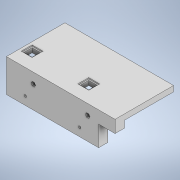
# Autodesk Inventor part: side_bumper
Saved by Autodesk Inventor 2020 (Build 240168000, 168)
## iProperties
Created: 2022-07-15
Part Number: side_bumper
Material: 일반
Document SubType Name: Modeling
Designer: SeungJin
Density: 1 g/cm^3
Appearance: 기본값
Author: SeungJin
Autodesk Inventor part; units mm, degrees
ref_plane "YZ Plane" through (0, 0, 0) normal (1, 0, 0) x (0, 1, 0)
sketch "스케치1" plane through (0, 0, 0) normal (0, 0, 1) x (1, 0, 0)
  line L0 (6, 0) -> (18, 0) projected
  line L1 (6, 0) -> (6, -540) projected
  line L2 (18, -540) -> (6, -540) projected
  line L3 (18, 0) -> (18, -540) projected
  line L4 (-12, 0) -> (0, 0) projected
  line L5 (-12, 0) -> (-12, -540) projected
  line L6 (0, -540) -> (-12, -540) projected
  line L7 (0, 0) -> (0, -540) projected
  line L8 (18, 22.5444) -> (18, 12.5098) projected
  line L9 (18, 12.5098) -> (18, -220) projected
  line L10 (-192.5399, 0) -> (-180.5399, 0) projected
  line L11 (-192.5399, 0) -> (-192.5399, -540) projected
  line L12 (-180.5399, -540) -> (-192.5399, -540) projected
  line L13 (-180.5399, 0) -> (-180.5399, -540) projected
  line L14 (-210.5399, 0) -> (-198.5399, 0) projected
  line L15 (-210.5399, 0) -> (-210.5399, -540) projected
  line L16 (-198.5399, -540) -> (-210.5399, -540) projected
  line L17 (-198.5399, 0) -> (-198.5399, -540) projected
  line L18 (18, 22.5444) -> (-210.5399, 22.5444)
  line L19 (-210.5399, 22.5444) -> (-210.5399, -37.4556)
  line L20 (-210.5399, -37.4556) -> (18, -37.4556)
  line L21 (18, -37.4556) -> (18, 22.5444)
  line L22 (18, 12.5444) -> (-210.5399, 12.5444)
  dimension "d0" = 60
  dimension "d1" = 10
  constraints: 10 end point, 3 point on line, 2 parallel, 2 perpendicular, 1 horizontal
  measures "d0" distance of L19.end L18.end
  measures "d1" distance between parallel lines of L22 L18
extrude "돌출1" add sketch "스케치1" along normal blind 10 and the other way blind 150 contours L22 L19 L18 L8
sketch "스케치2" plane through (-210.5399, 22.5444, 10) normal (0, 1, 0) x (1, 0, 0)
  line L0 (0, 0) -> (0, 160) projected
  line L1 (228.5399, 0) -> (0, 0) projected
  line L2 (228.5399, 160) -> (228.5399, 0) projected
  line L3 (0, 160) -> (228.5399, 160) projected
  circle A0 centre (-63.5, 111.3) radius 75.8469 projected
  line L4 (-155.5399, 160) -> (-155.5399, 55) projected
  line L5 (-139.3469, 111.3) -> (-155.5399, 111.3)
  line L6 (0, 0) -> (228.5399, 0) projected
  line L7 (30, 0) -> (30, 160)
  line L8 (0, 160) -> (0, 0) projected
  line L9 (30, 0) -> (0, 0)
  line L10 (0, 0) -> (0, 40)
  line L11 (0, 40) -> (30, 40)
  line L12 (30, 40) -> (30, 0)
  point P0 (210.5399, 10)
  point P1 (30, 40)
  dimension "d7" = 16.193
  dimension "d8" = 40
  dimension "d44" = 30
  constraints: 12 end point, 4 point on line, 3 perpendicular, 2 parallel, 1 horizontal, 1 horizontal alignment, 1 other
  measures "d7" distance of L5.start L5.end
  measures "d8" distance of L9.end L10.end
  measures "d44" distance between parallel lines of L7 L0
extrude "돌출2" cut sketch "스케치2" against normal through all contours L0 A0 L3 L7 L11 | L0 A0 picked at (1.772, 100.6693)
ref_plane "작업 평면1" through (-180.5399, 0, 0) normal (0, 0, 1) x (1, 0, 0)
sketch "스케치3" plane through (-180.5399, 0, 0) normal (0, 0, 1) x (1, 0, 0)
  line L0 (-30, 22.5444) -> (-30, 12.5444) projected
  line L1 (-30, 12.5444) -> (198.5399, 12.5444) projected
  line L2 (198.5399, 12.5444) -> (198.5399, 22.5444) projected
  line L3 (198.5399, 22.5444) -> (-30, 22.5444) projected
  line L4 (-30, 12.5444) -> (198.5399, 12.5444) projected
  line L5 (-30, 0) -> (-18, 0) projected
  line L6 (-30, 0) -> (-30, -540) projected
  line L7 (-18, -540) -> (-30, -540) projected
  line L8 (-18, 0) -> (-18, -540) projected
  line L9 (-12, 0) -> (0, 0) projected
  line L10 (-12, 0) -> (-12, -540) projected
  line L11 (0, -540) -> (-12, -540) projected
  line L12 (0, 0) -> (0, -540) projected
  line L13 (168.5399, 0) -> (180.5399, 0) projected
  line L14 (168.5399, 0) -> (168.5399, -540) projected
  line L15 (180.5399, -540) -> (168.5399, -540) projected
  line L16 (180.5399, 0) -> (180.5399, -540) projected
  line L17 (186.5399, 0) -> (198.5399, 0) projected
  line L18 (186.5399, 0) -> (186.5399, -540) projected
  line L19 (198.5399, -540) -> (186.5399, -540) projected
  line L20 (198.5399, 0) -> (198.5399, -540) projected
  line L21 (198.5399, 12.5444) -> (-30, 12.5444)
  line L22 (-30, 12.5444) -> (-30, -37.4556)
  line L23 (-30, -37.4556) -> (198.5399, -37.4556)
  line L24 (198.5399, -37.4556) -> (198.5399, 12.5444)
  dimension "d11" = 50
  constraints: 8 end point, 2 parallel, 1 horizontal, 1 perpendicular, 1 point on line
  measures "d11" distance of L22.end L21.end
extrude "돌출3" add sketch "스케치3" along normal blind 10 contours L1 L24 L17 L18 L23 L16 L13 L14 L12 L9 L10 L8 L5 L22 | L5 L8 L23 L6 | L20 L23 L18 L17 | L10 L9 L12 L23 | L23 L14 L13 L16
ref_plane "작업 평면2" through (-12, -260, -30) normal (0, 0, -1) x (0, 1, 0)
sketch "스케치4" plane through (-180.5399, 0, 0) normal (0, 0, -1) x (-1, 0, 0)
  line L0 (-180.5399, -260) -> (-168.5399, -260)
  line L1 (-168.5399, 0) -> (-168.5399, -260)
  line L2 (-180.5399, 0) -> (-168.5399, 0)
  line L3 (-180.5399, 0) -> (-180.5399, -260)
  line L4 (-198.5399, -260) -> (-186.5399, -260)
  line L5 (-186.5399, 0) -> (-186.5399, -260)
  line L6 (-198.5399, 0) -> (-186.5399, 0)
  line L7 (-198.5399, 0) -> (-198.5399, -260)
  line L8 (0, 12.5444) -> (0, 22.5444)
  line L9 (0, 22.5444) -> (-198.5399, 22.5444)
  line L10 (-198.5399, 22.5444) -> (-198.5399, 12.5444)
  line L11 (-198.5399, 12.5444) -> (0, 12.5444)
  line L12 (30, 12.5444) -> (0, 12.5444)
  line L13 (30, 22.5444) -> (30, 12.5444)
  line L14 (0, 22.5444) -> (30, 22.5444)
  line L15 (0, 22.5444) -> (0, 12.5444)
  line L16 (18, -260) -> (30, -260)
  line L17 (30, 0) -> (30, -260)
  line L18 (18, 0) -> (30, 0)
  line L19 (18, 0) -> (18, -260)
  line L20 (0, -260) -> (12, -260)
  line L21 (12, 0) -> (12, -260)
  line L22 (0, 0) -> (12, 0)
  line L23 (0, 0) -> (0, -260)
  line L24 (-198.5399, 0) -> (30, 0)
  line L25 (30, 0) -> (30, 12.5444)
  line L26 (30, 12.5444) -> (-198.5399, 12.5444)
  line L27 (-198.5399, 12.5444) -> (-198.5399, 0)
  line L28 (30, 12.5444) -> (30, -37.4556)
  line L29 (-198.5399, 12.5444) -> (30, 12.5444)
  line L30 (-198.5399, -37.4556) -> (-198.5399, 12.5444)
  line L31 (30, -37.4556) -> (-198.5399, -37.4556)
  line L32 (-198.5399, 0) -> (30, 0)
  line L33 (30, 0) -> (30, -37.4556)
  line L34 (30, -37.4556) -> (-198.5399, -37.4556)
  line L35 (-198.5399, -37.4556) -> (-198.5399, 0)
  line L36 (30, -37.4556) -> (-198.5399, -37.4556)
  line L37 (-99.27, 0) -> (-69.27, 0)
  line L38 (-69.27, 0) -> (-69.27, -37.4556)
  line L39 (-69.27, -37.4556) -> (-99.27, -37.4556)
  line L40 (-99.27, -37.4556) -> (-99.27, 0)
  line L41 (-99.27, 0) -> (-69.27, -37.4556) construction
  line L42 (-69.27, 0) -> (-99.27, -37.4556) construction
  line L43 (0, 0) -> (0, 12.5444)
  point P0 (-84.27, -18.7278)
  point P1 (0, -37.4556)
  point P2 (-168.5399, -37.4556)
extrude "돌출4" add sketch "스케치4" along normal blind 60 contours L1 L24 L40 L31 | L24 L6 L27 L11 L43 L2 | L40 L24 L38 L31 | L38 L24 L23 L31
sketch "스케치7" plane through (-180.5399, 0, 0) normal (0, 0, -1) x (-1, 0, 0)
  line L0 (0, -260) -> (12, -260) projected
  line L1 (12, 0) -> (12, -260) projected
  line L2 (0, 0) -> (12, 0) projected
  line L3 (0, 0) -> (0, -260) projected
  line L4 (18, -260) -> (30, -260) projected
  line L5 (30, 0) -> (30, -260) projected
  line L6 (18, 0) -> (30, 0) projected
  line L7 (18, 0) -> (18, -260) projected
  line L8 (30, 12.5444) -> (0, 12.5444) projected
  line L9 (30, 22.5444) -> (30, 12.5444) projected
  line L10 (0, 22.5444) -> (30, 22.5444) projected
  line L11 (0, 22.5444) -> (0, 12.5444) projected
  line L12 (-198.5399, 12.5444) -> (0, 12.5444) projected
  line L13 (0, 12.5444) -> (30, 12.5444)
  line L14 (30, 12.5444) -> (30, 0)
  line L15 (30, 0) -> (0, 0)
  line L16 (0, 0) -> (0, 12.5444)
  point P0 (-180.5399, 0)
  constraints: 8 end point, 2 parallel, 1 horizontal, 1 perpendicular
extrude "돌출7" add sketch "스케치7" along normal blind 30 contours L16 L8 L14 L6 L15 L2
sketch "스케치9" plane through (-210.5399, 22.5444, 10) normal (0, 1, 0) x (1, 0, 0)
  line L0 (30, 40) -> (0, 40) projected
  line L1 (0, 0) -> (0, 40) projected
  line L2 (228.5399, 0) -> (0, 0) projected
  line L3 (228.5399, 160) -> (228.5399, 0) projected
  line L4 (30, 160) -> (228.5399, 160) projected
  line L5 (30, 160) -> (30, 40) projected
  line L6 (30, 160) -> (30, 40) projected
  line L7 (228.5399, 75) -> (30, 75)
  line L8 (30, 75) -> (30, 95)
  line L9 (30, 95) -> (228.5399, 95)
  line L10 (228.5399, 95) -> (228.5399, 75)
  line L11 (158.5399, 75) -> (138.5399, 75)
  line L12 (138.5399, 75) -> (138.5399, 95)
  line L13 (138.5399, 95) -> (158.5399, 95)
  line L14 (158.5399, 95) -> (158.5399, 75)
  line L15 (158.5399, 75) -> (138.5399, 95) construction
  line L16 (138.5399, 75) -> (158.5399, 95) construction
  line L17 (55, 75) -> (35, 75)
  line L18 (35, 75) -> (35, 95)
  line L19 (35, 95) -> (55, 95)
  line L20 (55, 95) -> (55, 75)
  line L21 (55, 75) -> (35, 95) construction
  line L22 (35, 75) -> (55, 95) construction
  point P0 (210.5399, 10)
  point P1 (148.5399, 85)
  point P2 (45, 85)
  point P3 (55, 75)
  point P4 (55, 95)
  point P5 (35, 75)
  point P6 (158.5399, 75)
  point P7 (138.5399, 75)
  point P8 (148.5399, 85)
  point P9 (228.5399, 85)
  point P10 (45, 85)
  point P11 (30, 85)
  dimension "d45" = 20
  dimension "d46" = 65
  dimension "d48" = 80
  dimension "d49" = 20
  dimension "d50" = 15
  dimension "d101" = 20
  constraints: 32 end point, 8 midpoint, 6 parallel, 4 point on line, 3 horizontal, 3 perpendicular, 2 horizontal alignment
  measures "d45" distance of L7.end L8.end
  measures "d46" distance between parallel lines of L4 L9
  measures "d48" distance from line of point (148.54, 85) L3
  measures "d49" distance of L18.end L19.end
  measures "d50" distance from line of L5 point (45, 85)
  measures "d101" distance of L11.start L11.end
extrude "돌출8" cut sketch "스케치9" against normal blind 2 contours L18 L9 L20 L7 | L12 L9 L14 L7
sketch "스케치10" plane through (-210.5399, 20.5444, 10) normal (0, 1, 0) x (1, 0, 0)
  line L0 (138.5399, 75) -> (138.5399, 95) projected
  line L1 (158.5399, 75) -> (138.5399, 75) projected
  line L2 (158.5399, 95) -> (158.5399, 75) projected
  line L3 (138.5399, 95) -> (158.5399, 95) projected
  line L4 (55, 75) -> (35, 75) projected
  line L5 (55, 95) -> (55, 75) projected
  line L6 (35, 95) -> (55, 95) projected
  line L7 (35, 75) -> (35, 95) projected
  line L8 (156.0399, 77.5) -> (141.0399, 77.5)
  line L9 (141.0399, 77.5) -> (141.0399, 92.5)
  line L10 (141.0399, 92.5) -> (156.0399, 92.5)
  line L11 (156.0399, 92.5) -> (156.0399, 77.5)
  line L12 (156.0399, 77.5) -> (141.0399, 92.5) construction
  line L13 (141.0399, 77.5) -> (156.0399, 92.5) construction
  line L14 (52.5, 77.5) -> (37.5, 77.5)
  line L15 (37.5, 77.5) -> (37.5, 92.5)
  line L16 (37.5, 92.5) -> (52.5, 92.5)
  line L17 (52.5, 92.5) -> (52.5, 77.5)
  line L18 (52.5, 77.5) -> (37.5, 92.5) construction
  line L19 (37.5, 77.5) -> (52.5, 92.5) construction
  point P0 (210.5399, 10)
  point P1 (148.5399, 85)
  point P2 (45, 85)
  dimension "d53" = 15
  dimension "d54" = 15
  dimension "d55" = 15
  dimension "d56" = 15
  constraints: 24 end point, 4 midpoint, 4 parallel, 2 horizontal, 2 perpendicular
  measures "d53" distance of L9.end L10.end
  measures "d54" distance of L8.end L9.end
  measures "d55" distance of L15.end L16.end
  measures "d56" distance of L14.end L15.end
extrude "돌출9" cut sketch "스케치10" against normal through all contours L8 L9 L10 L11 | L14 L15 L16 L17
sketch "스케치11" plane through (-180.5399, 0, -60) normal (0, 0, -1) x (-1, 0, 0)
  line L0 (0, 12.5444) -> (0, 22.5444) projected
  line L1 (0, 22.5444) -> (-198.5399, 22.5444) projected
  line L2 (-198.5399, 22.5444) -> (-198.5399, 12.5444) projected
  line L3 (-198.5399, 12.5444) -> (0, 12.5444) projected
  line L4 (-168.5399, -37.4556) -> (0, -37.4556) projected
  line L5 (-198.5399, 12.5444) -> (0, 12.5444) projected
  line L6 (-198.5399, 12.5444) -> (-198.5399, 0) projected
  line L7 (-198.5399, 0) -> (-168.5399, 0) projected
  line L8 (-168.5399, 0) -> (-168.5399, -37.4556) projected
  line L9 (0, -37.4556) -> (0, 12.5444) projected
  line L10 (-198.5399, 12.5444) -> (0, 12.5444)
  line L11 (0, 12.5444) -> (0, -5.4556)
  line L12 (0, -5.4556) -> (-198.5399, -5.4556)
  line L13 (-198.5399, -5.4556) -> (-198.5399, 12.5444)
  line L14 (-128.5399, 12.5444) -> (-108.5399, 12.5444)
  line L15 (-108.5399, 12.5444) -> (-108.5399, -5.4556)
  line L16 (-108.5399, -5.4556) -> (-128.5399, -5.4556)
  line L17 (-128.5399, -5.4556) -> (-128.5399, 12.5444)
  line L18 (-128.5399, 12.5444) -> (-108.5399, -5.4556) construction
  line L19 (-108.5399, 12.5444) -> (-128.5399, -5.4556) construction
  line L20 (-25, 12.5444) -> (-5, 12.5444)
  line L21 (-5, 12.5444) -> (-5, -5.4556)
  line L22 (-5, -5.4556) -> (-25, -5.4556)
  line L23 (-25, -5.4556) -> (-25, 12.5444)
  line L24 (-25, 12.5444) -> (-5, -5.4556) construction
  line L25 (-5, 12.5444) -> (-25, -5.4556) construction
  circle A0 centre (-34.635, -22.4556) radius 3.6
  circle A1 centre (-133.9049, -22.4556) radius 3.6
  line L26 (-36.7134, -26.0556) -> (-38.7919, -22.4556)
  line L27 (-38.7919, -22.4556) -> (-36.7134, -18.8556)
  line L28 (-36.7134, -18.8556) -> (-32.5565, -18.8556)
  line L29 (-32.5565, -18.8556) -> (-30.4781, -22.4556)
  line L30 (-30.4781, -22.4556) -> (-32.5565, -26.0556)
  line L31 (-32.5565, -26.0556) -> (-36.7134, -26.0556)
  line L32 (-135.9834, -26.0556) -> (-138.0619, -22.4556)
  line L33 (-138.0619, -22.4556) -> (-135.9834, -18.8556)
  line L34 (-135.9834, -18.8556) -> (-131.8265, -18.8556)
  line L35 (-131.8265, -18.8556) -> (-129.748, -22.4556)
  line L36 (-129.748, -22.4556) -> (-131.8265, -26.0556)
  line L37 (-131.8265, -26.0556) -> (-135.9834, -26.0556)
  line L38 (0, -37.4556) -> (0, 12.5444) projected
  point P0 (-180.5399, 0)
  point P1 (-118.5399, 3.5444)
  point P2 (-15, 3.5444)
  point P3 (-148.5399, 3.5444)
  point P4 (-49.27, 3.5444)
  point P5 (-34.635, -26.0556)
  point P6 (-133.9049, -26.0556)
  dimension "d71" = 7.2
  dimension "d59" = 18
  dimension "d60" = 20
  dimension "d61" = 20
  dimension "d63" = 80
  dimension "d64" = 20
  dimension "d69" = 15
  dimension "d72" = 7.2
  constraints: 56 end point, 6 midpoint, 6 parallel, 4 coincident, 4 point on line, 3 horizontal, 3 perpendicular, 1 centre point, 1 vertical alignment, 28 other
  measures "d59" distance of L10.end L11.end
  measures "d60" distance of L15.end L16.end
  measures "d61" distance of L21.end L22.end
  measures "d63" distance from line of L6 point (-118.54, 3.544)
  measures "d64" distance from line of point (-148.54, 3.544) L8
  measures "d69" distance from line of L4 point (-34.635, -22.456)
  measures "d72" diameter of A1
sketch "스케치12" plane through (-210.5399, 22.5444, 10) normal (0, 1, 0) x (1, 0, 0)
  line L0 (35, 95) -> (55, 95) projected
  line L1 (55, 95) -> (55, 75) projected
  line L2 (55, 75) -> (35, 75) projected
  line L3 (35, 75) -> (35, 95) projected
  line L4 (138.5399, 75) -> (138.5399, 95) projected
  line L5 (138.5399, 95) -> (158.5399, 95) projected
  line L6 (158.5399, 95) -> (158.5399, 75) projected
  line L7 (158.5399, 75) -> (138.5399, 75) projected
  line L8 (30, 40) -> (0, 40) projected
  line L9 (0, 0) -> (0, 40) projected
  line L10 (228.5399, 0) -> (0, 0) projected
  line L11 (228.5399, 160) -> (228.5399, 0) projected
  line L12 (30, 160) -> (228.5399, 160) projected
  line L13 (30, 160) -> (30, 40) projected
  line L14 (228.5399, 0) -> (0, 0)
  line L15 (0, 0) -> (0, 53)
  line L16 (0, 53) -> (228.5399, 53)
  line L17 (228.5399, 53) -> (228.5399, 0)
  point P0 (210.5399, 10)
  point P1 (228.5399, 53)
  point P2 (30, 53)
  dimension "d66" = 53
  constraints: 8 end point, 2 parallel, 1 horizontal, 1 perpendicular
  measures "d66" distance of L14.end L15.end
extrude "돌출10" cut sketch "스케치12" against normal through all contours L13 L16 L11 L10 L9 L8
extrude "돌출11" cut sketch "스케치11" against normal blind 12 contours A0 | A0 L29 L30 | A0 L28 L29 | L30 L31 A0 | A0 L27 L28 | L31 L26 A0 | A0 L26 L27 | A1 | A1 L35 L36 | A1 L34 L35 | L36 L37 A1 | A1 L33 L34 | L37 L32 A1 | A1 L32 L33
sketch "스케치13" plane through (-180.5399, 0, -48) normal (0, 0, -1) x (-1, 0, 0)
  line L0 (-36.7134, -18.8556) -> (-32.5565, -18.8556) projected
  line L1 (-38.7919, -22.4556) -> (-36.7134, -18.8556) projected
  line L2 (-36.7134, -26.0556) -> (-38.7919, -22.4556) projected
  line L3 (-32.5565, -26.0556) -> (-36.7134, -26.0556) projected
  line L4 (-30.4781, -22.4556) -> (-32.5565, -26.0556) projected
  line L5 (-32.5565, -18.8556) -> (-30.4781, -22.4556) projected
  line L6 (-135.9834, -26.0556) -> (-138.0619, -22.4556) projected
  line L7 (-131.8265, -26.0556) -> (-135.9834, -26.0556) projected
  line L8 (-129.748, -22.4556) -> (-131.8265, -26.0556) projected
  line L9 (-131.8265, -18.8556) -> (-129.748, -22.4556) projected
  line L10 (-135.9834, -18.8556) -> (-131.8265, -18.8556) projected
  line L11 (-138.0619, -22.4556) -> (-135.9834, -18.8556) projected
  point P0 (-180.5399, 0)
  point P1 (-34.635, -22.4556)
  point P2 (-133.9049, -22.4556)
hole "구멍1" at (-145.9049, -22.4556, -48) at (-46.635, -22.4556, -48) direction (0, 0, 1) diameter 4.5 end through all clearance for "Hex Head Cap Screw ISO 24017" size "M4" standard "ISO"
sketch "스케치14" plane through (-180.5399, 22.5444, -43) normal (0, 0, 1) x (1, 0, 0)
  circle A0 centre (34.635, -45) radius 2.25 projected
  circle A1 centre (133.9049, -45) radius 2.25 projected
  line L0 (168.5399, -60) -> (0, -60) projected
  line L1 (198.5399, -22.5444) -> (168.5399, -22.5444) projected
  line L2 (168.5399, -22.5444) -> (168.5399, -60) projected
  line L3 (198.5399, 0) -> (198.5399, -22.5444) projected
  line L4 (0, 0) -> (198.5399, 0) projected
  line L5 (0, -60) -> (0, 0) projected
  line L6 (0, 0) -> (198.5399, 0) projected
  line L7 (198.5399, 0) -> (198.5399, -22.5444) projected
  line L8 (0, 0) -> (198.5399, 0)
  line L9 (198.5399, 0) -> (198.5399, -22.5444)
  line L10 (0, -22.5444) -> (0, 0)
  line L11 (5, -22.5444) -> (25, -22.5444)
  line L12 (25, -22.5444) -> (25, 0)
  line L13 (25, 0) -> (5, 0)
  line L14 (5, 0) -> (5, -22.5444)
  line L15 (5, -22.5444) -> (25, 0) construction
  line L16 (25, -22.5444) -> (5, 0) construction
  line L17 (108.5399, -22.5444) -> (128.5399, -22.5444)
  line L18 (128.5399, -22.5444) -> (128.5399, 0)
  line L19 (128.5399, 0) -> (108.5399, 0)
  line L20 (108.5399, 0) -> (108.5399, -22.5444)
  line L21 (108.5399, -22.5444) -> (128.5399, 0) construction
  line L22 (128.5399, -22.5444) -> (108.5399, 0) construction
  line L23 (0, -60) -> (0, -10) projected
  line L24 (0, -28) -> (198.5399, -28)
  line L25 (0, -10) -> (198.5399, -10)
  line L26 (25, -28) -> (25, -22.5444)
  line L27 (69.27, -22.5444) -> (69.27, -60) projected
  line L28 (69.27, -28) -> (69.27, -10)
  line L29 (168.5399, -22.5444) -> (168.5399, -60) projected
  line L30 (168.5399, -28) -> (168.5399, -10)
  line L31 (128.5399, -22.5444) -> (128.5399, -28)
  line L32 (25, -22.5444) -> (0, -22.5444)
  line L33 (198.5399, -22.5444) -> (168.5399, -22.5444)
  line L34 (128.5399, -22.5444) -> (69.27, -22.5444)
  circle A2 centre (49.27, -19) radius 3.6
  circle A3 centre (148.5399, -19) radius 3.6
  line L35 (47.1915, -22.6) -> (45.113, -19)
  line L36 (45.113, -19) -> (47.1915, -15.4)
  line L37 (47.1915, -15.4) -> (51.3484, -15.4)
  line L38 (51.3484, -15.4) -> (53.4269, -19)
  line L39 (53.4269, -19) -> (51.3484, -22.6)
  line L40 (51.3484, -22.6) -> (47.1915, -22.6)
  line L41 (146.4615, -22.6) -> (144.383, -19)
  line L42 (144.383, -19) -> (146.4615, -15.4)
  line L43 (146.4615, -15.4) -> (150.6184, -15.4)
  line L44 (150.6184, -15.4) -> (152.6968, -19)
  line L45 (152.6968, -19) -> (150.6184, -22.6)
  line L46 (150.6184, -22.6) -> (146.4615, -22.6)
  point P0 (180.5399, -22.5444)
  point P1 (15, -11.2722)
  point P2 (118.5399, -11.2722)
  point P3 (49.27, -22.6)
  point P4 (148.5399, -22.6)
  dimension "d90" = 7.2
  dimension "d82" = 20
  dimension "d83" = 15
  dimension "d84" = 20
  dimension "d85" = 80
  dimension "d86" = 28
  dimension "d87" = 10
  dimension "d88" = 20
  dimension "d89" = 20
  constraints: 72 end point, 16 point on line, 8 parallel, 6 midpoint, 5 horizontal, 5 perpendicular, 4 coincident, 2 vertical alignment, 1 vertical, 30 other
  measures "d82" distance of L13.end L12.end
  measures "d83" distance from line of point (15, -11.272) L5
  measures "d84" distance of L19.end L18.end
  measures "d85" distance from line of point (118.54, -11.272) L3
  measures "d86" distance between parallel lines of L4 L24
  measures "d87" distance between parallel lines of L4 L25
  measures "d88" distance from line of point (49.27, -19) L28
  measures "d89" distance from line of point (148.54, -19) L30
extrude "돌출12" cut sketch "스케치14" against normal blind 12 contours A2 | A2 L38 L39 | A2 L37 L38 | L39 L40 A2 | A2 L36 L37 | L40 L35 A2 | A2 L35 L36 | A3 | A3 L44 L45 | A3 L43 L44 | L45 L46 A3 | A3 L42 L43 | L46 L41 A3 | A3 L41 L42
sketch "스케치15" plane through (-180.5399, 22.5444, -55) normal (0, 0, 1) x (1, 0, 0)
  line L0 (51.3484, -22.6) -> (47.1915, -22.6) projected
  line L1 (53.4269, -19) -> (51.3484, -22.6) projected
  line L2 (51.3484, -15.4) -> (53.4269, -19) projected
  line L3 (47.1915, -15.4) -> (51.3484, -15.4) projected
  line L4 (45.113, -19) -> (47.1915, -15.4) projected
  line L5 (47.1915, -22.6) -> (45.113, -19) projected
  line L6 (150.6184, -15.4) -> (152.6968, -19) projected
  line L7 (146.4615, -15.4) -> (150.6184, -15.4) projected
  line L8 (144.383, -19) -> (146.4615, -15.4) projected
  line L9 (146.4615, -22.6) -> (144.383, -19) projected
  line L10 (150.6184, -22.6) -> (146.4615, -22.6) projected
  line L11 (152.6968, -19) -> (150.6184, -22.6) projected
  point P0 (180.5399, -22.5444)
  point P1 (49.27, -19)
  point P2 (148.5399, -19)
hole "구멍2" at (-131.27, 3.5444, -55) at (-32, 3.5444, -55) direction (0, 0, -1) diameter 4.5 end through all clearance for "Hex Head Cap Screw ISO 24017" size "M4" standard "ISO"
